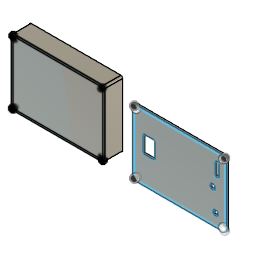
smp3d (Autodesk Fusion 360 design; units mm, degrees)
part number: 2025-10-23-16-47-43-892
part number: 2025-10-23-16-48-02-880
Autodesk Fusion 360 part; units mm, degrees
sketch "Sketch1" plane through (0, 0, 0) normal (0, 1, 0) x (1, 0, 0) in component "sketch1"
  line L0 (2, 0) -> (98, 0)
  line L1 (100, -2) -> (100, -68)
  line L2 (98, -70) -> (2, -70)
  line L3 (0, -68) -> (0, -2)
  line L4 (0, 2) -> (100, 2)
  line L5 (102, 0) -> (102, -70)
  line L6 (100, -72) -> (0, -72)
  line L7 (-2, -70) -> (-2, 0)
  arc A0 (-2, -70) -> (0, -72) centre (0, -70) ccw
  arc A1 (0, 2) -> (-2, 0) centre (0, 0) ccw
  arc A2 (102, 0) -> (100, 2) centre (100, 0) ccw
  arc A3 (100, -72) -> (102, -70) centre (100, -70) ccw
  arc A4 (0, -68) -> (2, -70) centre (2, -68) ccw
  arc A5 (2, 0) -> (0, -2) centre (2, -2) ccw
  arc A6 (100, -2) -> (98, 0) centre (98, -2) ccw
  arc A7 (98, -70) -> (100, -68) centre (98, -68) ccw
  point P0 (100, 0)
  point P1 (0, -70)
  dimension "d1" = 100
  dimension "d2" = 70
  dimension "d4" = 2
  dimension "d5" = 2
  constraint horizontal L0
  constraint vertical L1
  constraint horizontal L2
  constraint vertical L3
  constraint coincident A1.centre origin
  constraint tangent L6 A0
  constraint tangent L7 A0
  constraint tangent L7 A1
  constraint tangent L4 A1
  constraint equal A0 A1
  constraint tangent L4 A2
  constraint tangent L5 A2
  constraint equal A0 A2
  constraint tangent L5 A3
  constraint tangent L6 A3
  constraint equal A0 A3
  constraint coincident P1 L2
  constraint coincident P1 L3
  constraint tangent L2 A4
  constraint tangent L3 A4
  constraint coincident A1.centre L3
  constraint coincident A1.centre L0
  constraint tangent L3 A5
  constraint tangent L0 A5
  constraint equal A4 A5
  constraint coincident P0 L0
  constraint coincident P0 L1
  constraint tangent L0 A6
  constraint tangent L1 A6
  constraint equal A4 A6
  constraint tangent L1 A7
  constraint tangent L2 A7
  constraint equal A4 A7
  measures "d1" distance of A1.centre P0
  measures "d2" distance of A1.centre A0.centre
  measures "d4" radius of A0
  measures "d5" radius of A4
extrude "Extrude1" add sketch "Sketch1" along normal blind 2 contours L0 L1 L2 L3 A4 A5 A6 A7 makes body 1 in component "sketch1"
extrude "Extrude2" add sketch "Sketch1" along normal blind 2 bodies 1 in component "sketch1"
extrude "Extrude3" add sketch "Sketch1" along normal blind 20 bodies 1 in component "sketch1"
sketch "Sketch2" plane through (0, 0, 0) normal (0, 1, 0) x (1, 0, 0) in component "sketch1"
  line L0 (137, -70) -> (233.713, -70)
  line L1 (235.713, -68) -> (235.713, -2)
  line L2 (233.713, 0) -> (137, 0)
  line L3 (135, -2) -> (135, -68)
  line L4 (235.713, 2) -> (135, 2)
  line L5 (133, 0) -> (133, -70)
  line L6 (135, -72) -> (235.713, -72)
  line L7 (237.713, -70) -> (237.713, 0)
  arc A0 (133, -70) -> (135, -72) centre (135, -70) ccw
  arc A1 (135, 2) -> (133, 0) centre (135, 0) ccw
  arc A2 (237.713, 0) -> (235.713, 2) centre (235.713, 0) ccw
  arc A3 (235.713, -72) -> (237.713, -70) centre (235.713, -70) ccw
  arc A4 (135, -68) -> (137, -70) centre (137, -68) ccw
  arc A5 (137, 0) -> (135, -2) centre (137, -2) ccw
  arc A6 (235.713, -2) -> (233.713, 0) centre (233.713, -2) ccw
  arc A7 (233.713, -70) -> (235.713, -68) centre (233.713, -68) ccw
  line L8 (144.6546, -47.9172) -> (157.6546, -47.9172)
  line L9 (157.6546, -47.9172) -> (157.6546, -28.9172)
  line L10 (157.6546, -28.9172) -> (144.6546, -28.9172)
  line L11 (144.6546, -28.9172) -> (144.6546, -47.9172)
  line L12 (219.3175, -38.1174) -> (224.3175, -38.1174)
  line L13 (224.3175, -38.1174) -> (224.3175, -33.1174)
  line L14 (224.3175, -33.1174) -> (219.3175, -33.1174)
  line L15 (219.3175, -33.1174) -> (219.3175, -38.1174)
  line L16 (222.7027, -14.343) -> (227.7027, -14.343)
  line L17 (227.7027, -14.343) -> (227.7027, -9.343)
  line L18 (227.7027, -9.343) -> (222.7027, -9.343)
  line L19 (222.7027, -9.343) -> (222.7027, -14.343)
  line L20 (224.8697, -62.0573) -> (228.8697, -62.0573)
  line L21 (228.8697, -62.0573) -> (228.8697, -47.0573)
  line L22 (228.8697, -47.0573) -> (224.8697, -47.0573)
  line L23 (224.8697, -47.0573) -> (224.8697, -62.0573)
  point P0 (135, -70)
  point P1 (235.713, -70)
  point P2 (135, 0)
  dimension "d12" = 100.713
  dimension "d13" = 70
  dimension "d15" = 2
  dimension "d16" = 2
  dimension "d21" = 13
  dimension "d22" = 19
  dimension "d23" = 5
  dimension "d24" = 5
  dimension "d25" = 5
  dimension "d26" = 5
  dimension "d33" = 4
  dimension "d34" = 15
  constraint horizontal L0
  constraint vertical L1
  constraint horizontal L2
  constraint vertical L3
  constraint tangent L6 A0
  constraint tangent L5 A0
  constraint tangent L5 A1
  constraint tangent L4 A1
  constraint equal A0 A1
  constraint tangent L4 A2
  constraint tangent L7 A2
  constraint equal A0 A2
  constraint tangent L7 A3
  constraint tangent L6 A3
  constraint equal A0 A3
  constraint coincident P0 L0
  constraint coincident P0 L3
  constraint tangent L0 A4
  constraint tangent L3 A4
  constraint coincident P2 L3
  constraint coincident P2 L2
  constraint tangent L3 A5
  constraint tangent L2 A5
  constraint equal A4 A5
  constraint tangent L2 A6
  constraint tangent L1 A6
  constraint equal A4 A6
  constraint coincident P1 L1
  constraint coincident P1 L0
  constraint tangent L1 A7
  constraint tangent L0 A7
  constraint equal A4 A7
  constraint horizontal L8
  constraint vertical L9
  constraint horizontal L10
  constraint vertical L11
  constraint horizontal L12
  constraint vertical L13
  constraint horizontal L14
  constraint vertical L15
  constraint horizontal L16
  constraint vertical L17
  constraint horizontal L18
  constraint vertical L19
  constraint horizontal L20
  constraint vertical L21
  constraint horizontal L22
  constraint vertical L23
  measures "d12" distance of P0 A3.centre
  measures "d13" distance of P0 P2
  measures "d15" radius of A0
  measures "d16" radius of A4
  measures "d21" distance of L8.start L8.end
  measures "d22" distance of L8.start L10.end
  measures "d23" distance of L12.start L12.end
  measures "d24" distance of L12.start L14.end
  measures "d25" distance of L16.start L16.end
  measures "d26" distance of L16.start L18.end
  measures "d33" distance of L20.start L20.end
  measures "d34" distance of L20.start L22.end
extrude "Extrude4" add sketch "Sketch2" along normal blind 2 separate body contours L0 L1 L2 L3 A4 A5 A6 A7 | L8 L9 L10 L11 | L12 L13 L14 L15 | L16 L17 L18 L19 | L20 L21 L22 L23 makes body 2 in component "sketch1"
extrude "Extrude5" add sketch "Sketch2" along normal blind 2 contours L4 L5 L6 L7 A0 A1 A2 A3 bodies 2 in component "sketch1"
extrude "Extrude6" cut sketch "Sketch2" along normal blind 2 contours L8 L9 L10 L11 bodies 2 in component "sketch1"
extrude "Extrude7" cut sketch "Sketch2" along normal blind 2 contours L12 L13 L14 L15 bodies 2 in component "sketch1"
extrude "Extrude8" cut sketch "Sketch2" along normal blind 2 contours L16 L17 L18 L19 bodies 2 in component "sketch1"
extrude "Extrude9" cut sketch "Sketch2" along normal blind 2 contours L20 L21 L22 L23 bodies 2 in component "sketch1"
component "sketch1" placed x (1, 0, 0) y (0, 1, 0) z (0, 0, 1) at (0, 0, 0)
